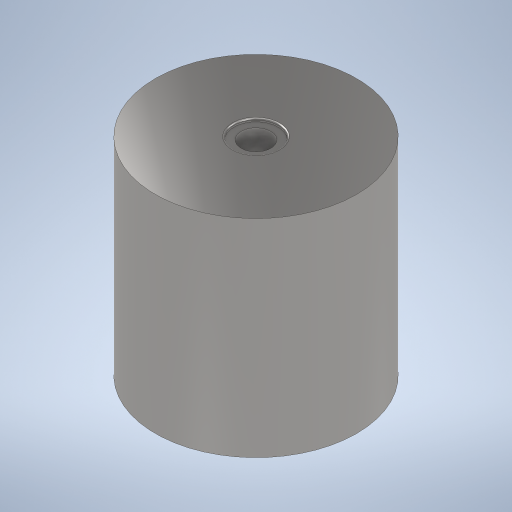
# Autodesk Inventor part: top
Saved by Autodesk Inventor 2024 (Build 280153020, 153B)
## iProperties
Created: 2023-06-12
Part Number: top
Material: Steel, Mild
Document SubType Name: Modeling
Designer: OKESH
Density: 7.85 g/cm^3
Appearance: Semi-Polished
Author: OKESH
Autodesk Inventor part; units mm, degrees
ref_plane "YZ Plane" through (0, 0, 0) normal (1, 0, 0) x (0, 1, 0)
ref_plane "XZ Plane" through (0, 0, 0) normal (0, 1, 0) x (-1, 0, 0)
ref_plane "XY Plane" through (0, 0, 0) normal (0, 0, 1) x (1, 0, 0)
sketch "Sketch1" plane through (0, 0, 0) normal (0, 1, 0) x (-1, 0, 0)
  circle A0 centre (0, 0) radius 33.995
  circle A1 centre (0, 0) radius 5.005
  dimension "d0" = 67.99
  dimension "d1" = 10.01
  constraints: 2 centre point, 2 coincident
  measures "d0" diameter of A0
  measures "d1" diameter of A1
extrude "Extrusion1" add sketch "Sketch1" along normal blind 70
sketch "Sketch2" plane through (0, 0, 0) normal (0, -1, 0) x (1, 0, 0)
  circle A0 centre (0, 0) radius 5.005 projected
  circle A1 centre (0, 0) radius 10.005
  dimension "d4" = 20.01
  constraints: 1 centre point, 1 coincident
  measures "d4" diameter of A1
extrude "Extrusion2" cut sketch "Sketch2" against normal blind 50
sketch "Sketch3" plane through (0, 70, 0) normal (0, 1, 0) x (1, 0, 0)
  circle A0 centre (0, 0) radius 7.5
  dimension "d7" = 15
  constraints: 1 centre point, 1 coincident
  measures "d7" diameter of A0
extrude "Extrusion3" cut sketch "Sketch3" against normal blind 1
fillet "Fillet1" radius 0.5 1 edges at (-7.5, 70, 0)
body "Solid1"
